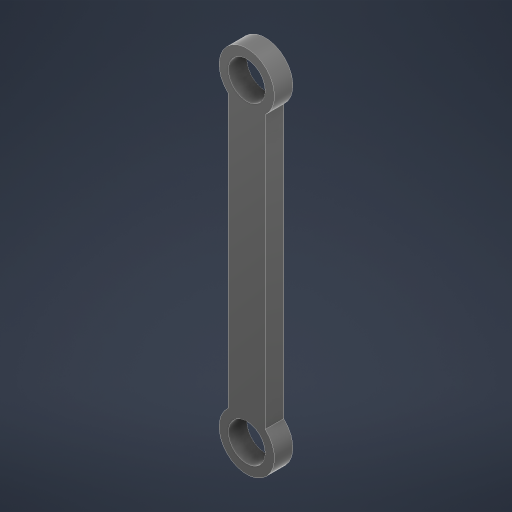
# Autodesk Inventor part: FP V2 Lengan Serok
Saved by Autodesk Inventor 2023.6 (Build 276521000, 521)
## iProperties
Created: 2026-02-12
Part Number: FP V2 Lengan Serok
Material: Aluminum 6061
Document SubType Name: Modeling
Designer: user
Density: 2.7 g/cm^3
Appearance: Smooth - Black
Author: user
Autodesk Inventor part; units mm, degrees
ref_plane "YZ Plane" through (0, 0, 0) normal (1, 0, 0) x (0, 1, 0)
ref_plane "XZ Plane" through (0, 0, 0) normal (0, 1, 0) x (-1, 0, 0)
ref_plane "XY Plane" through (0, 0, 0) normal (0, 0, 1) x (1, 0, 0)
sketch "Sketch1" plane through (0, 0, 0) normal (0, 0, 1) x (1, 0, 0)
  line L0 (0, 0) -> (-5, 0)
  line L1 (-5, 0) -> (-5, 98.0902)
  line L2 (-3.75, 100) -> (-1.25, 100)
  line L3 (0, 0) -> (5, 0)
  line L4 (5, 0) -> (5, 98.0902)
  line L5 (2.5, 195) -> (0, 195)
  circle A0 centre (0, 92.5) radius 7.5
  circle A1 centre (0, 92.5) radius 5
  line L6 (0, 195) -> (0, 188.836)
  line L7 (5, 0) -> (5, 50)
  line L8 (5, 50) -> (-5, 50)
  circle A2 centre (0, 7.5) radius 7.5
  circle A3 centre (0, 7.5) radius 5
  line L9 (0, 0) -> (0, 25.2031)
  point P0 (-2.5, 0)
  point P1 (5, 86.9098)
  point P2 (-5, 86.9098)
  point P3 (-5, 13.0902)
  point P4 (5, 13.0902)
  dimension "d1" = 100
  dimension "d4" = 15
  dimension "d5" = 10
  dimension "d6" = 50
  dimension "d9" = 5
  dimension "d10" = 5
  constraints: 20 end point, 4 centre point, 4 point on line, 3 parallel, 3 perpendicular, 2 coincident, 2 horizontal, 2 point on circle, 2 symmetric about line, 1 midpoint, 1 tangent, 1 vertical, 2 other
  measures "d1" distance from line of point (-2.5, 0) L2
  measures "d4" diameter of A0
  measures "d5" diameter of A1
  measures "d6" distance of L3.end L7.end
  measures "d9" distance between parallel lines of L4 L9
  measures "d10" distance between parallel lines of L1 L9
extrude "Extrusion1" add sketch "Sketch1" along normal blind 5 contours L9 A3 L4 A2 | A2 L1 A3 L9 | A2 L1 | L4 A2 | L1 A2 L9 A3 | L1 L8 L4 A2 | A3 L9 A2 L4 | L1 A0 L4 L8 | A0 L1 | L1 A1 L4 A0 | L1 A0 L4 A1 | L4 A0
body "Solid1"
